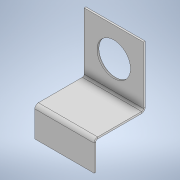
# Autodesk Inventor part: Soporte Sensor Inductivo
Saved by Autodesk Inventor 2021 (Build 250183000, 183)
## iProperties
Created: 2021-08-02
Part Number: Soporte Sensor Inductivo
Material: Generic
Document SubType Name: Sheet Metal
Designer: Nelson
Density: 1 g/cm^3
Sheet Metal Rule: Default_mm
Appearance: Default
Author: Nelson
Autodesk Inventor part; units mm, degrees
ref_plane "YZ Plane" through (0, 0, 0) normal (1, 0, 0) x (0, 1, 0)
ref_plane "XZ Plane" through (0, 0, 0) normal (0, 1, 0) x (-1, 0, 0)
ref_plane "XY Plane" through (0, 0, 0) normal (0, 0, 1) x (1, 0, 0)
sketch "Sketch1" plane through (0, 0, 0) normal (0, 0, 1) x (1, 0, 0)
  line L0 (0, 0) -> (30, 0)
  line L1 (30, 0) -> (30, 15)
  line L2 (30, 15) -> (0, 15)
  line L3 (0, 15) -> (0, 0)
  dimension "d0" = 15
  dimension "d1" = 30
  measures "d0" distance of L0.end L1.end
  measures "d1" distance of L1.end L2.end
extrude "Plate1" add sketch "Sketch1" against normal blind 0.9
sketch "Sketch2" plane through (30, 14.1, 0) normal (0, 1, 0) x (-1, 0, 0)
  line L0 (30, 0) -> (0, 0)
  line L1 (0, 0) -> (0, -25.9)
  line L2 (0, -25.9) -> (30, -25.9)
  line L3 (30, -25.9) -> (30, 0)
  constraints: 6 end point, 1 horizontal, 1 perpendicular, 1 vertical
edge flange "Flange1" height 25.9 angle 90 thickness 0.9 bend radius 0.9 thickness toward (0, 1, 0) relief straight relief width 0.9 relief depth 0.45 edges at (15, 15, -0.9) wall of the first edge with corners at (0, 14.1, 0) (30, 14.1, 0) (30, 14.1, -25.9) (0, 14.1, -25.9)
bend "Bend1"
corner "Corner1"
sketch "Sketch3" plane through (0, 14.1, -25) normal (0, 0, -1) x (-1, 0, 0)
  line L0 (-30, 0) -> (0, 0)
  line L1 (0, 0) -> (0, 30.9)
  line L2 (0, 30.9) -> (-30, 30.9)
  line L3 (-30, 30.9) -> (-30, 0)
  constraints: 6 end point, 1 horizontal, 1 perpendicular, 1 vertical
edge flange "Flange2" height 30.9 angle 90 thickness 0.9 bend radius 0.9 thickness toward (0, 0, -1) relief straight relief width 0.9 relief depth 0.45 edges at (15, 15, -25.9) wall of the first edge with corners at (30, 14.1, -25) (0, 14.1, -25) (0, 45, -25) (30, 45, -25)
bend "Bend2"
corner "Corner2"
sketch "Sketch4" plane through (30, 45, -25.9) normal (0, 0, -1) x (-1, 0, 0)
  line L0 (30, 0) -> (30, -29.1) projected
  line L1 (0, 0) -> (30, 0) projected
  point P0 (30, -45)
  point P1 (15, -15)
  dimension "d23" = 15
  dimension "d24" = 15
  measures "d23" distance from line of L0 point (15, -15)
  measures "d24" distance from line of L1 point (15, -15)
hole "Hole1" at (15, 30, -25.9) direction (0, 0, 1) diameter 16.9175 end through all thread size "M18x1" class "6H" standard "ISO Metric profile"
equation "\"d2\" = Thickness"
equation "\"d3\" = BendReliefWidth"
equation "\"d4\" = BendReliefDepth"
equation "\"d5\" = MinimumRemnant"
equation "\"d6\" = TransitionRadius"
equation "\"d9\" = BendRadius"
equation "\"d10\" = CornerReliefSize"
equation "\"d11\" = GapSize"
equation "\"d12\" = JacobiRadiusSize"
equation "\"d13\" = BendReliefWidth"
equation "\"d14\" = BendReliefDepth"
equation "\"d15\" = MinimumRemnant"
equation "\"d16\" = TransitionRadius"
equation "\"d19\" = BendRadius"
equation "\"d20\" = CornerReliefSize"
equation "\"d21\" = GapSize"
equation "\"d22\" = JacobiRadiusSize"
equation "\"d24\" = d23"
equation "\"BendRadius\" = Thickness"
equation "\"BendReliefWidth\" = Thickness"
equation "\"BendReliefDepth\" = 0.5 * Thickness"
equation "\"CornerReliefSize\" = 4 * Thickness"
equation "\"MinimumRemnant\" = 2 * Thickness"
equation "\"TransitionRadius\" = BendRadius"
equation "\"JacobiRadiusSize\" = BendRadius"
equation "\"GapSize\" = Thickness"
equation "\"Thickness\" = 0.9"
body "Solid1"
